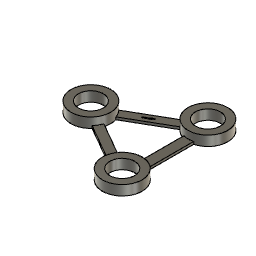
Model 24 (Autodesk Fusion 360 design; units mm, degrees)
Autodesk Fusion 360 part; units mm, degrees
sketch "Sketch1" plane through (0, 0, 0) normal (0, 0, 1) x (1, 0, 0)
  circle A0 centre (0, 0) radius 25
  circle A1 centre (0, 0) radius 40
  circle A2 centre (149.9956, 86.6) radius 25
  circle A3 centre (149.9956, 86.6) radius 40
  circle A4 centre (149.9956, -86.6) radius 25
  circle A5 centre (149.9956, -86.6) radius 40
  line L0 (149.9956, 46.6) -> (149.9956, -46.6) construction
  line L1 (111.8461, -74.5744) -> (29.4892, -27.0256)
  line L2 (111.8461, 74.5744) -> (29.4892, 27.0256)
  line L3 (139.9956, 47.8702) -> (139.9956, -47.8702)
  line L4 (120.5064, -59.5744) -> (38.1495, -12.0256)
  line L5 (34.641, -20) -> (115.3546, -66.6) construction
  line L6 (120.5064, 59.5744) -> (38.1495, 12.0256)
  line L7 (34.641, 20) -> (115.3546, 66.6) construction
  line L8 (159.9956, 47.8702) -> (159.9956, -47.8702)
  line L9 (40, 0) -> (159.9956, 0) construction
  line L10 (40, 0) -> (159.9956, 0) construction
  dimension "d1" = 50
  dimension "d2" = 80
  dimension "d3" = 173.2
  dimension "d6" = 173.2
  dimension "d7" = 50
  dimension "d8" = 80
  dimension "d9" = 50
  dimension "d10" = 80
  constraint coincident A0.centre A1.centre
  constraint concentric A2 A3
  constraint concentric A4 A5
  constraint coincident A1 L2.end
  constraint coincident A1 L6.end
  constraint coincident A1 L7.start
  constraint coincident A1 L4.end
  constraint coincident A1 L5.start
  constraint coincident A1 L1.end
  constraint coincident A5 L8.end
  constraint coincident A5 L3.end
  constraint coincident A5 L4.start
  constraint coincident A5 L1.start
  constraint coincident A5 L5.end
  constraint coincident A3 L6.start
  constraint coincident A3 L2.start
  constraint coincident A3 L7.end
  constraint coincident A3 L3.start
  constraint coincident A3 L8.start
  constraint coincident A5 L0.end
  constraint coincident A1 L9.start
  constraint coincident A3 L0.start
  constraint coincident L8 L9.end
  measures "d1" diameter of A0
  measures "d2" diameter of A1
  measures "d3" distance of A0.centre A2.centre
  measures "d6" distance of A0.centre A4.centre
  measures "d7" diameter of A2
  measures "d8" diameter of A3
  measures "d9" diameter of A4
  measures "d10" diameter of A5
extrude "Extrude1" add sketch "Sketch1" along normal blind 5 contours A1 A3 L2 L6 | A1 A5 L1 L4 | A3 A5 L3 L8 makes body 1 at (61.9995, 34.6765, 0) makes body 2 at (146.6355, -15.5333, 0) makes body 3 at (88.9651, -50.2451, 0)
extrude "Extrude2" add sketch "Sketch1" along normal blind 20 separate body contours A1 | A3 | A5 makes body 4 at (39.8012, 3.9827, 13.3333) makes body 5 at (189.7968, 82.6173, 6.6667) makes body 6 at (189.7968, -90.5827, 6.6667)
ref_plane "WorkPlane1" through (74.9978, 43.3, 5) normal (0, 0, 1) x (1, 0, 0)
sketch "Sketch2" plane through (74.9978, 43.3, 5) normal (0, 0, 1) x (1, 0, 0)
  line L0 (-20.4729, -19.1403) -> (24.4449, 6.5131) construction
  line L1 (24.4449, 6.5131) -> (17.8785, 18.0106) construction
  line L2 (17.8785, 18.0106) -> (-27.0393, -7.6429) construction
  line L3 (-27.0393, -7.6429) -> (-20.4729, -19.1403) construction
  text T0 "enes şahin" font "Arial" height 3 align centre middle in box 51.7272 x 13.2404 at (-20.4729, -19.1403) x (0.868358, 0.495937) y (-0.495937, 0.868358) spacing 1
extrude "Extrude3" add sketch "Sketch2" along normal blind 0.5 text T0 bodies 1
